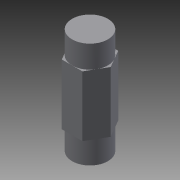
# Autodesk Inventor part: Hex Shaft for E gear box
Saved by Autodesk Inventor 2015 (Build 190159000, 159)
## iProperties
Created: 2015-02-14
Part Number: Hex Shaft for E gear box
Material: Generic
Document SubType Name: Modeling
Designer: whitaus15
Density: 1 g/cm^3
Appearance: Default
Author: whitaus15
Autodesk Inventor part; units mm, degrees
ref_plane "YZ Plane" through (0, 0, 0) normal (1, 0, 0) x (0, 1, 0)
ref_plane "XZ Plane" through (0, 0, 0) normal (0, 1, 0) x (-1, 0, 0)
ref_plane "XY Plane" through (0, 0, 0) normal (0, 0, 1) x (1, 0, 0)
sketch "Sketch1" plane through (0, 0, 0) normal (0, 1, 0) x (-1, 0, 0)
  line L0 (7.3323, 0) -> (3.6662, -6.35)
  line L1 (3.6662, -6.35) -> (-3.6662, -6.35)
  line L2 (-3.6662, -6.35) -> (-7.3323, 0)
  line L3 (-7.3323, 0) -> (-3.6662, 6.35)
  line L4 (-3.6662, 6.35) -> (3.6662, 6.35)
  line L5 (3.6662, 6.35) -> (7.3323, 0)
  line L6 (7.3323, 0) -> (0, 0)
  line L7 (0, 0) -> (0, -3.7196)
  dimension "d0" = 90
  dimension "d1" = 12.7
  constraints: 16 end point, 1 coincident, 1 vertical, 13 other
  measures "d0" angle of L7 L6
  measures "d1" distance between parallel lines of L1 L4
extrude "Extrusion1" add sketch "Sketch1" along normal blind 37.465
ref_plane "Work Plane2" through (0, 18.7325, 0) normal (0, 1, 0) x (1, 0, 0)
sketch "Sketch3" plane through (0, 37.465, 0) normal (0, 1, 0) x (1, 0, 0)
  circle A0 centre (0, 0) radius 6.35
  line L0 (-3.6662, 6.35) -> (-7.3323, 0) projected
  line L1 (-3.6662, 6.35) -> (-7.3323, 0) projected
  line L2 (-7.3323, 0) -> (-3.6662, -6.35) projected
  line L3 (-3.6662, -6.35) -> (3.6662, -6.35) projected
  line L4 (3.6662, -6.35) -> (7.3323, 0) projected
  line L5 (7.3323, 0) -> (3.6662, 6.35) projected
  line L6 (3.6662, 6.35) -> (-3.6662, 6.35) projected
  dimension "d7" = 12.7
  constraints: 1 centre point, 1 coincident
  measures "d7" diameter of A0
extrude "Extrusion3" cut sketch "Sketch3" against normal blind 8 contours A0 L5 L4 | A0 L6 L5 | L4 L3 A0 | A0 L0 L6 | L3 L2 A0 | A0 L2 L0
mirror "Mirror2" about plane through (0, 18.7325, 0) normal (0, 1, 0) of "Extrusion3"
body "Solid1"
